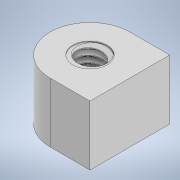
# Autodesk Inventor part: Bending Wire Fixture
Saved by Autodesk Inventor 2022.2 (Build 262287000, 287)
## iProperties
Created: 2022-08-14
Part Number: Bending Wire Fixture
Material: Generic
Document SubType Name: Modeling
Designer: Ilewicz
Density: 1 g/cm^3
Appearance: Default
Author: Ilewicz
Autodesk Inventor part; units mm, degrees
ref_plane "YZ Plane" through (0, 0, 0) normal (1, 0, 0) x (0, 1, 0)
ref_plane "XZ Plane" through (0, 0, 0) normal (0, 1, 0) x (-1, 0, 0)
ref_plane "XY Plane" through (0, 0, 0) normal (0, 0, 1) x (1, 0, 0)
sketch "Sketch3" plane through (0, 3.7, 0) normal (1, 0, 0) x (0, 0, 1)
  line L0 (1.075, 0) -> (1.075, 3.7)
  line L1 (1.075, 3.7) -> (0.7784, 3.7)
  line L2 (0.7784, 3.7) -> (0.7784, 0)
  line L3 (0.7784, 0) -> (1.075, 0)
  line L4 (0, -0.74) -> (0, 4.44) projected
  constraints: 8 end point
revolve "Revolution1" add sketch "Sketch3" angle 360 about axis through (0, 3.7, 0) along (0, -1, 0)
sketch "Sketch2" plane through (0, 3.7, 1.075) normal (-1, 0, 0) x (0, -1, 0)
  line L0 (-0.2334, -0.0204) -> (-0.2001, -0.0204) construction
  line L1 (0.0332, -0.2765) -> (-0.0001, -0.3406) construction
  line L2 (-0.4001, -0.3406) -> (-0.4334, -0.2765) construction
  line L3 (-0.1668, -0.0204) -> (-0.2001, 0.0436) construction
  line L4 (-0.2001, 0.0436) -> (-0.2334, -0.0204) construction
  line L5 (-0.4001, -0.3406) -> (-0.3668, -0.2765) construction
  line L6 (-0.1668, -0.0204) -> (-0.0334, -0.2765)
  line L7 (-0.4334, -0.2765) -> (-0.3668, -0.2765) construction
  arc A0 (-0.4334, -0.2765) -> (-0.4001, -0.2968) centre (-0.4001, -0.2592) ccw construction
  line L8 (0.0332, -0.2765) -> (-0.0334, -0.2765) construction
  line L9 (-0.4001, -0.3406) -> (-0.4001, -0.2765) construction
  line L10 (-0.0001, -0.3406) -> (-0.0001, -0.2765) construction
  line L11 (-0.2001, 0.0436) -> (-0.2001, -0.0002) construction
  line L12 (-0.4001, -0.2968) -> (-0.0001, -0.2968)
  arc A1 (-0.4001, -0.2968) -> (-0.3668, -0.2765) centre (-0.4001, -0.2592) ccw
  line L13 (-0.0334, -0.2765) -> (-0.0001, -0.3406) construction
  line L14 (-0.3668, -0.2765) -> (-0.2334, -0.0204)
  line L15 (-0.0001, -0.0002) -> (-0.0001, 0.0177)
  line L16 (-0.0001, 0.0177) -> (-0.0001, -0.0002)
  line L17 (-0.0001, -0.0002) -> (0.0334, -0.0002)
  arc A2 (-0.0334, -0.2765) -> (-0.0001, -0.2968) centre (-0.0001, -0.2592) ccw
  arc A3 (-0.0001, -0.2968) -> (0.0332, -0.2765) centre (-0.0001, -0.2592) ccw construction
  arc A4 (-0.2001, -0.0002) -> (-0.2334, -0.0204) centre (-0.2001, -0.0377) ccw
  arc A5 (-0.1668, -0.0204) -> (-0.2001, -0.0002) centre (-0.2001, -0.0377) ccw
  line L18 (-0.2001, -0.0002) -> (-0.2001, -0.0204) construction
  line L19 (-0.2001, -0.0204) -> (-0.1668, -0.0204) construction
  dimension "d10" = 55
  dimension "d11" = 0.064
  dimension "d12" = 0.064
  dimension "Sketch2_ThreadOffset" = 0
  dimension "Sketch2_MajorRadius" = 0.2966
  dimension "d15" = 0.4
  dimension "Sketch2_MinorRadius" = 0
  constraints: 40 end point, 12 point on circle, 10 parallel, 8 tangent, 6 centre point, 6 collinear, 2 midpoint, 2 point on line, 1 horizontal, 1 perpendicular, 3 other
  measures "d10" angle of L6 L14
  measures "d11" distance of L3.end L0.end
  measures "d12" distance of L1.end L10.end
  measures "Sketch2_ThreadOffset" distance between parallel lines of L15 L10
  measures "Sketch2_MajorRadius" distance from line of L12 L15.start
  measures "d15" distance from line of L1.end L9
  measures "Sketch2_MinorRadius" distance edge to line of A5 L17
coil "Coil1" sketch "Sketch2" operation cut axis through (0, 3.7, 0) along (0, -1, 0) pitch 0.4004 turns 11.238761 hand right
sketch "Sketch5" plane through (0, 0, 0) normal (0, 1, 0) x (-1, 0, 0)
  arc A0 (0, -2.5) -> (0, 2.5) centre (0, 0) ccw
  line L0 (0, 2.5) -> (-2.5, 2.5)
  line L1 (-2.5, 2.5) -> (-2.5, -2.5)
  line L2 (-2.5, -2.5) -> (0, -2.5)
  circle A1 centre (0, 0) radius 1.075
  point P0 (0, 0)
  dimension "d30" = 2.5
  dimension "d31" = 2.5
  dimension "d32" = 5
  constraints: 6 end point, 2 centre point, 2 coincident, 2 perpendicular, 2 point on circle, 1 horizontal
  measures "d30" radius of A0
  measures "d31" distance of L0.start L0.end
  measures "d32" distance of L0.end L1.end
extrude "Extrusion2" add sketch "Sketch5" along normal blind 3.75
equation "\"d10\" = d17"
equation "\"d11\" = 0.160083 * Sketch2_Pitch"
equation "\"d12\" = 0.160083 * Sketch2_Pitch"
equation "\"d15\" = Sketch2_Pitch"
equation "\"d30\" = d33"
equation "\"d31\" = d33"
equation "\"d32\" = 2 * d33"
equation "\"d17\" = 55deg"
equation "\"Sketch2_Pitch\" = 0.4"
equation "\"d33\" = 2.5"
body "Solid2"
body "Solid1"
